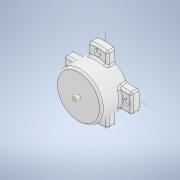
# Autodesk Inventor part: Base
Saved by Autodesk Inventor 2021 (Build 250183000, 183)
## iProperties
Created: 2021-03-25
Part Number: Base
Material: ABS 플라스틱
Document SubType Name: Modeling
Designer: jglee
Mass: 957.385 g
Surface Area: 663.299 cm^2
Volume: 903.193 cm^3
Density: 1.06 g/cm^3
Appearance: 매끄러움 - 흰색
Author: jglee
Autodesk Inventor part; units mm, degrees
ref_plane "YZ Plane" through (0, 0, 0) normal (1, 0, 0) x (0, 1, 0)
ref_plane "XZ Plane" through (0, 0, 0) normal (0, 1, 0) x (-1, 0, 0)
ref_plane "XY Plane" through (0, 0, 0) normal (0, 0, 1) x (1, 0, 0)
sketch "스케치2" plane through (0, 0, 0) normal (0, 0, 1) x (1, 0, 0)
  circle A0 centre (0, 0) radius 90
  dimension "d3" = 180
  constraints: 1 centre point, 1 coincident
  measures "d3" diameter of A0
extrude "돌출2" add sketch "스케치2" along normal blind 20
sketch "스케치3" plane through (0, 0, 20) normal (0, 0, 1) x (1, 0, 0)
  circle A0 centre (0, 0) radius 60
  dimension "d6" = 120
  constraints: 1 centre point, 1 coincident
  measures "d6" diameter of A0
extrude "돌출3" add sketch "스케치3" along normal blind 50
sketch "스케치4" plane through (0, 0, 20) normal (0, 0, 1) x (1, 0, 0)
  circle A0 centre (0, 0) radius 60 projected
  circle A1 centre (0, 0) radius 60 projected
  circle A2 centre (0, 0) radius 90 projected
  line L0 (-25, -100) -> (25, -100)
  line L1 (25, -100) -> (25, 100)
  line L2 (25, 100) -> (-25, 100)
  line L3 (-25, 100) -> (-25, -100)
  line L4 (100, -25) -> (100, 25)
  line L5 (100, 25) -> (-100, 25)
  line L6 (-100, 25) -> (-100, -25)
  line L7 (-100, -25) -> (100, -25)
  line L8 (25, 100) -> (-25, 100)
  line L9 (-25, 100) -> (-25, -100)
  line L10 (-25, -100) -> (25, -100)
  line L11 (25, -100) -> (25, 100)
  line L12 (-100, 25) -> (-100, -25)
  line L13 (-100, -25) -> (100, -25)
  line L14 (100, -25) -> (100, 25)
  line L15 (100, 25) -> (-100, 25)
  point P0 (0, 100)
  point P1 (-25, 0)
  point P2 (-100, 0)
  point P3 (0, -25)
  point P4 (0, -100)
  point P5 (25, 0)
  point P6 (100, 0)
  point P7 (0, 25)
  point P8 (-54.5436, -25)
  point P9 (-86.4581, -25)
  point P10 (-25, -86.4581)
  point P11 (-25, -54.5436)
  point P12 (-86.4581, 25)
  point P13 (-54.5436, 25)
  point P14 (-25, 54.5436)
  point P15 (-25, 86.4581)
  point P16 (54.5436, 25)
  point P17 (86.4581, 25)
  point P18 (25, 86.4581)
  point P19 (25, 54.5436)
  point P20 (86.4581, -25)
  point P21 (54.5436, -25)
  point P22 (25, -54.5436)
  point P23 (25, -86.4581)
  dimension "d9" = 200
  dimension "d10" = 50
  dimension "d13" = 360
  constraints: 32 end point, 2 midpoint, 2 parallel, 1 horizontal, 1 horizontal alignment, 1 perpendicular, 1 vertical alignment, 41 other
  measures "d9" distance between parallel lines of L0 L2
  measures "d10" distance between parallel lines of L3 L1
extrude "돌출4" cut sketch "스케치4" against normal up to next contours A0 L1 A2 L5 | L7 A2 L1 A0 | A0 L5 A2 L3 | L3 A2 L7 A0
fillet "모깎기1" radius 5 34 edges at (-60, 0, 70) (0, -60, 20) (58.62, 12.7943, 20) (58.62, -12.7943, 20) (0, 60, 20) (-60, 0, 20) (-90, 0, 20) (0, 90, 20) (90, 0, 20) (0, -90, 20) (25, -70.5008, 20) (70.5008, -25, 20) (-25, -70.5008, 20) (-70.5008, -25, 20) (-70.5008, 25, 20) (-25, 70.5008, 20) (25, 70.5008, 20) (70.5008, 25, 20) (25, -54.5436, 10) (54.5436, -25, 10) (-25, -54.5436, 10) (-54.5436, -25, 10) (-54.5436, 25, 10) (-25, 54.5436, 10) (25, 54.5436, 10) (54.5436, 25, 10) (-86.4581, 25, 10) (-86.4581, -25, 10) (-25, -86.4581, 10) (25, -86.4581, 10) (86.4581, -25, 10) (86.4581, 25, 10) (25, 86.4581, 10) (-25, 86.4581, 10)
sketch "스케치5" plane through (0, 0, 70) normal (0, 0, 1) x (1, 0, 0)
  circle A0 centre (0, 0) radius 5
  dimension "d18" = 10
  constraints: 1 centre point, 1 coincident
  measures "d18" diameter of A0
extrude "돌출5" add sketch "스케치5" along normal blind 10
sketch "스케치6" plane through (0, 0, 20) normal (0, 0, 1) x (1, 0, 0)
  arc A0 (-61.8466, 20) -> (-61.8466, -20) centre (0, 0) ccw projected
  line L0 (-82.6136, 20) -> (-61.8466, 20) projected
  arc A1 (-82.6136, 20) -> (-82.6136, -20) centre (0, 0) ccw projected
  line L1 (-61.8466, -20) -> (-82.6136, -20) projected
  arc A2 (61.8466, -20) -> (61.8466, 20) centre (0, 0) ccw projected
  line L2 (82.6136, -20) -> (61.8466, -20) projected
  arc A3 (82.6136, -20) -> (82.6136, 20) centre (0, 0) ccw projected
  line L3 (61.8466, 20) -> (82.6136, 20) projected
  arc A4 (20, 61.8466) -> (-20, 61.8466) centre (0, 0) ccw projected
  line L4 (20, 82.6136) -> (20, 61.8466) projected
  arc A5 (20, 82.6136) -> (-20, 82.6136) centre (0, 0) ccw projected
  line L5 (-20, 61.8466) -> (-20, 82.6136) projected
  arc A6 (-20, -61.8466) -> (20, -61.8466) centre (0, 0) ccw projected
  line L6 (-20, -82.6136) -> (-20, -61.8466) projected
  arc A7 (-20, -82.6136) -> (20, -82.6136) centre (0, 0) ccw projected
  line L7 (20, -61.8466) -> (20, -82.6136) projected
  circle A8 centre (0, 0) radius 5 projected
  circle A9 centre (0, 0) radius 55 projected
  circle A10 centre (-75, 0) radius 5
  circle A11 centre (0, -75) radius 5
  circle A12 centre (75, 0) radius 5
  circle A13 centre (0, 75) radius 5
  dimension "d21" = 10
  dimension "d22" = 75
  dimension "d25" = 360
  constraints: 4 centre point, 9 other
  measures "d21" diameter of A10
  measures "d22" distance of A10.centre point (0, 0)
extrude "돌출6" cut sketch "스케치6" against normal up to next contours A10 | A11 | A12 | A13
sketch "스케치7" plane through (0, 0, 20) normal (0, 0, 1) x (1, 0, 0)
  circle A0 centre (-75, 0) radius 5 projected
  arc A1 (-61.8466, 20) -> (-61.8466, -20) centre (0, 0) ccw projected
  line L0 (-82.6136, 20) -> (-61.8466, 20) projected
  arc A2 (-82.6136, 20) -> (-82.6136, -20) centre (0, 0) ccw projected
  line L1 (-61.8466, -20) -> (-82.6136, -20) projected
  circle A3 centre (0, 75) radius 5 projected
  arc A4 (20, 61.8466) -> (-20, 61.8466) centre (0, 0) ccw projected
  line L2 (20, 82.6136) -> (20, 61.8466) projected
  arc A5 (20, 82.6136) -> (-20, 82.6136) centre (0, 0) ccw projected
  line L3 (-20, 61.8466) -> (-20, 82.6136) projected
  circle A6 centre (75, 0) radius 5 projected
  arc A7 (61.8466, -20) -> (61.8466, 20) centre (0, 0) ccw projected
  line L4 (82.6136, -20) -> (61.8466, -20) projected
  arc A8 (82.6136, -20) -> (82.6136, 20) centre (0, 0) ccw projected
  line L5 (61.8466, 20) -> (82.6136, 20) projected
  circle A9 centre (0, -75) radius 5 projected
  arc A10 (-20, -61.8466) -> (20, -61.8466) centre (0, 0) ccw projected
  line L6 (-20, -82.6136) -> (-20, -61.8466) projected
  arc A11 (-20, -82.6136) -> (20, -82.6136) centre (0, 0) ccw projected
  line L7 (20, -61.8466) -> (20, -82.6136) projected
  circle A12 centre (0, 0) radius 5 projected
  circle A13 centre (0, 0) radius 55 projected
  circle A14 centre (-75, 0) radius 8
  circle A15 centre (0, -75) radius 8
  circle A16 centre (75, 0) radius 8
  circle A17 centre (0, 75) radius 8
  dimension "d29" = 16
  dimension "d32" = 360
  constraints: 4 centre point, 1 coincident, 9 other
  measures "d29" diameter of A14
extrude "돌출7" cut sketch "스케치7" against normal blind 4 contours A0 | A3 | A6 | A9 | A14 | A15 | A16 | A17
